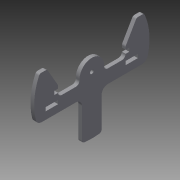
# Autodesk Inventor part: Endplate 072313
Saved by Autodesk Inventor 2015 (Build 190159000, 159)
## iProperties
Created: 2013-05-25
Part Number: Endplate 072313
Material: Generic
Document SubType Name: Modeling
Designer: Eric
Density: 1 g/cm^3
Appearance: Default
Author: Eric
Autodesk Inventor part; units mm, degrees
ref_plane "YZ Plane" through (0, 0, 0) normal (1, 0, 0) x (0, 1, 0)
ref_plane "XZ Plane" through (0, 0, 0) normal (0, 1, 0) x (-1, 0, 0)
ref_plane "XY Plane" through (0, 0, 0) normal (0, 0, 1) x (1, 0, 0)
sketch "Sketch1" plane through (0, 0, 0) normal (1, 0, 0) x (0, 1, 0)
  line L0 (-46.6154, -6) -> (46.6154, -6) construction
  line L1 (-37.5, -6) -> (-27.5, -6)
  line L2 (-27.5, -6) -> (-27.5, -9)
  line L3 (-27.5, -9) -> (-37.5, -9)
  line L4 (-37.5, -9) -> (-37.5, -6)
  line L5 (27.5, -6) -> (37.5, -6)
  line L6 (37.5, -6) -> (37.5, -9)
  line L7 (37.5, -9) -> (27.5, -9)
  line L8 (27.5, -9) -> (27.5, -6)
  arc A0 (10, 0) -> (-10, 0) centre (0, 0) ccw
  circle A1 centre (0, 0) radius 1.5
  line L9 (-35.955, 19) -> (-27.9019, 5.0517)
  line L10 (27.9019, 5.0517) -> (35.955, 19)
  line L11 (-8, -44.5982) -> (-8, -20)
  line L12 (8, -44.5982) -> (8, -20)
  arc A2 (-6.2667, -46.5803) -> (6.2667, -46.5803) centre (0, 0) ccw
  line L13 (-25, -39.7995) -> (25, -39.7995) construction
  line L14 (40.7922, -15) -> (13, -15)
  line L15 (-40.8058, -15) -> (-13, -15)
  arc A3 (45.6484, -11.1905) -> (43.0762, 18.8) centre (0, 0) ccw
  line L16 (-46.7846, 0) -> (47, 0) construction
  arc A4 (-45.5561, -11.5602) -> (-40.8058, -15) centre (-40.8058, -10) ccw
  arc A5 (40.7922, -15) -> (45.6484, -11.1905) centre (40.7922, -10) ccw
  arc A6 (-43.0762, 18.8) -> (-45.5561, -11.5602) centre (0, 0) ccw
  line L17 (-41.2432, 20) -> (-37.687, 20)
  line L18 (37.687, 20) -> (41.2432, 20)
  arc A7 (-41.2432, 20) -> (-43.0762, 18.8) centre (-41.2432, 18) ccw
  arc A8 (-35.955, 19) -> (-37.687, 20) centre (-37.687, 18) ccw
  arc A9 (43.0762, 18.8) -> (41.2432, 20) centre (41.2432, 18) ccw
  arc A10 (37.687, 20) -> (35.955, 19) centre (37.687, 18) ccw
  line L19 (-27.5, -1) -> (-30.5, -1)
  line L20 (-30.5, -1) -> (-30.5, 2)
  line L21 (-30.5, 2) -> (-27.5, 2)
  line L22 (27.5, -1) -> (30.5, -1)
  line L23 (30.5, -1) -> (30.5, 2)
  line L24 (30.5, 2) -> (27.5, 2)
  arc A11 (-8, -44.5982) -> (-6.2667, -46.5803) centre (-6, -44.5982) ccw
  arc A12 (6.2667, -46.5803) -> (8, -44.5982) centre (6, -44.5982) ccw
  line L25 (-27.5, 2) -> (-27.5, 3.5517)
  line L26 (27.5, 2) -> (27.5, 3.5517)
  line L27 (-27.5, -1) -> (-27.5, -1)
  line L28 (27.5, -1) -> (27.5, -1)
  line L29 (-10, 0) -> (-10, -1)
  line L30 (10, 0) -> (10, -1)
  line L31 (-24.5, -4) -> (-13, -4)
  line L32 (13, -4) -> (24.5, -4)
  arc A13 (-27.5, -1) -> (-24.5, -4) centre (-24.5, -1) ccw
  arc A14 (-27.5, 3.5517) -> (-27.9019, 5.0517) centre (-30.5, 3.5517) ccw
  arc A15 (-13, -4) -> (-10, -1) centre (-13, -1) ccw
  arc A16 (10, -1) -> (13, -4) centre (13, -1) ccw
  arc A17 (24.5, -4) -> (27.5, -1) centre (24.5, -1) ccw
  arc A18 (27.9019, 5.0517) -> (27.5, 3.5517) centre (30.5, 3.5517) ccw
  arc A19 (-8, -20) -> (-13, -15) centre (-13, -20) ccw
  arc A20 (13, -15) -> (8, -20) centre (13, -20) ccw
  point P0 (-42.5323, 20)
  point P1 (42.5323, 20)
  point P2 (-36.5323, 20)
  point P3 (36.5323, 20)
  point P4 (-26.14, 2)
  point P5 (26.14, 2)
  point P6 (-8, -10)
  point P7 (8, -10)
  point P8 (-45.4579, -15)
  point P9 (44.5421, -15)
  point P10 (-25.4579, -10)
  point P11 (8, -15)
  point P12 (-8, -15)
  point P13 (-8, -46.3141)
  point P14 (8, -46.3141)
  dimension "d3" = 10
  dimension "d4" = 3
  dimension "d5" = 10
  dimension "d6" = 3
  dimension "d105" = 50
  dimension "d116" = 6
  dimension "d122" = 8
  dimension "d123" = 8
  dimension "d131" = 47
  dimension "d137" = 5
  dimension "d141" = 6
  dimension "d142" = 120
  dimension "d143" = 6
  dimension "d144" = 120
  dimension "d145" = 2
  dimension "d146" = 3
  dimension "d147" = 3
  dimension "d148" = 5
  dimension "d149" = 3
  dimension "d150" = 3
  dimension "d151" = 5
  dimension "d154" = 47
  dimension "d155" = 10
  dimension "d156" = 2
  dimension "d159" = 20
  dimension "d160" = 20
  dimension "d162" = 3
  dimension "d163" = 15
  dimension "d164" = 15
  dimension "d167" = 30.5
  dimension "d168" = 30.5
  dimension "d169" = 3
  dimension "d170" = 3
  dimension "d171" = 27.5
  dimension "d172" = 27.5
  dimension "d173" = 5
  dimension "d174" = 11
  dimension "d175" = 11
  constraints: 66 end point, 49 point on circle, 33 tangent, 22 point on line, 21 centre point, 11 equal radius, 10 parallel, 10 perpendicular, 8 horizontal, 5 coincident, 2 vertical, 1 collinear, 1 horizontal alignment
  measures "d3" distance between parallel lines of L2 L4
  measures "d4" distance between parallel lines of L3 L0
  measures "d5" distance between parallel lines of L6 L8
  measures "d6" distance between parallel lines of L0 L7
  measures "d105" distance of L13.start L13.end
  measures "d116" distance from line of point (0, 0) L0
  measures "d122" distance from line of point (0, 0) L11
  measures "d123" distance from line of L12 point (0, 0)
  measures "d131" radius of A3
  measures "d137" radius of A4
  measures "d141" distance of point (-42.532, 20) point (-36.532, 20)
  measures "d142" angle of L9 L17
  measures "d143" distance of point (36.532, 20) point (42.532, 20)
  measures "d144" angle of L10 L18
  measures "d145" radius of A7
  measures "d146" distance of L19.start L19.end
  measures "d147" distance of L21.end L19.start
  measures "d148" distance between parallel lines of L1 L19
  measures "d149" distance of L22.start L22.end
  measures "d150" distance of L24.end L22.start
  measures "d151" distance between parallel lines of L5 L22
  measures "d154" radius of A2
  measures "d155" radius of A0
  measures "d156" radius of A11
  measures "d159" distance from line of point (0, 0) L17
  measures "d160" distance from line of L18 point (0, 0)
  measures "d162" radius of A13
  measures "d163" distance from line of point (0, 0) L15
  measures "d164" distance from line of L14 point (0, 0)
  measures "d167" distance from line of A2.centre L20
  measures "d168" distance from line of point (0, 0) L23
  measures "d169" distance of L19.end L20.end
  measures "d170" distance of L22.end L23.end
  measures "d171" distance from line of point (0, 0) L2
  measures "d172" distance from line of point (0, 0) L8
  measures "d173" radius of A19
  measures "d174" distance between parallel lines of L15 L31
  measures "d175" distance between parallel lines of L14 L32
extrude "Extrusion5" add sketch "Sketch1" along normal blind 3
body "Solid5"
